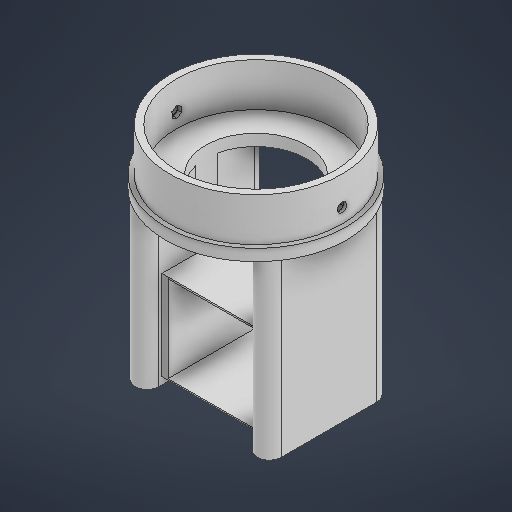
# Autodesk Inventor part: cam_mount0
Saved by Autodesk Inventor 2027 (Build 310192060, 192F)
## iProperties
Created: 2026-07-16
Part Number: cam_mount0
Material: Generic
Document SubType Name: Modeling
Designer: farde
Density: 1 g/cm^3
Appearance: Default
Author: farde
Autodesk Inventor part; units mm, degrees
ref_plane "YZ Plane" through (0, 0, 0) normal (1, 0, 0) x (0, 1, 0)
ref_plane "XZ Plane" through (0, 0, 0) normal (0, 1, 0) x (-1, 0, 0)
ref_plane "XY Plane" through (0, 0, 0) normal (0, 0, 1) x (1, 0, 0)
sketch "Sketch1" plane through (0, 0, 0) normal (0, 1, 0) x (-1, 0, 0)
  circle A0 centre (0, 0) radius 29.85
  circle A1 centre (0, 0) radius 27.5
  dimension "d0" = 59.7
  dimension "d1" = 55
  constraints: 2 centre point, 2 coincident
  measures "d0" diameter of A0
  measures "d1" diameter of A1
extrude "Extrusion1" add sketch "Sketch1" along normal blind 15
sketch "Sketch2" plane through (0, 0, 0) normal (0, 1, 0) x (-1, 0, 0)
  circle A0 centre (0, 0) radius 31.4135
  circle A1 centre (0, 0) radius 28.9404
  circle A2 centre (0, 0) radius 31.4135
  circle A3 centre (0, 0) radius 20.0919
  dimension "d6" = 40.1837
  constraints: 4 centre point, 4 coincident, 1 concentric
  measures "d6" diameter of A3
extrude "Extrusion2" add sketch "Sketch2" against normal blind 4 contours A0 | A1 | A3
sketch "Sketch3" plane through (0, -4, 0) normal (0, -1, 0) x (1, 0, 0)
  line L0 (21.2066, 16.5968) -> (21.2066, -16.5968) construction
  line L1 (17.0959, 16.5968) -> (17.0959, -16.5968)
  line L2 (25.3174, -16.5968) -> (25.3174, 16.5968)
  arc A0 (25.3174, 16.5968) -> (17.0959, 16.5968) centre (21.2066, 16.5968) ccw
  arc A1 (17.0959, -16.5968) -> (25.3174, -16.5968) centre (21.2066, -16.5968) ccw
  point P0 (0, 0)
  point P1 (21.2066, 0)
  dimension "d28" = 8.2215
  constraints: 8 end point, 4 point on circle, 4 tangent, 2 centre point, 1 midpoint, 1 parallel, 1 vertical
  measures "d28" distance between parallel lines of L1 L2
extrude "Extrusion3" add sketch "Sketch3" along normal blind 60
mirror "Mirror1" about plane through (0, 0, 0) normal (1, 0, 0) of "Extrusion3"
sketch "Sketch4" plane through (0, 0, 0) normal (0, 1, 0) x (1, 0, 0)
  circle A0 centre (0, 0) radius 17.5
  dimension "d11" = 35
  constraints: 1 centre point, 1 coincident
  measures "d11" diameter of A0
extrude "Extrusion4" cut sketch "Sketch4" against normal blind 60
sketch "Sketch5" plane through (17.0959, -64, -16.5968) normal (-1, 0, 0) x (0, 0, 1)
  line L0 (32.0968, 2.4749) -> (1.0968, 2.4749)
  line L1 (1.0968, 2.4749) -> (1.0968, 33.4749)
  line L2 (1.0968, 33.4749) -> (32.0968, 33.4749)
  line L3 (32.0968, 33.4749) -> (32.0968, 2.4749)
  line L4 (32.0968, 2.4749) -> (1.0968, 33.4749) construction
  line L5 (1.0968, 2.4749) -> (32.0968, 33.4749) construction
  point P0 (16.5968, 64)
  point P1 (16.5968, 17.9749)
  dimension "d12" = 31
  dimension "d13" = 31
  constraints: 12 end point, 2 midpoint, 2 parallel, 1 horizontal, 1 perpendicular
  measures "d12" distance of L1.end L2.end
  measures "d13" distance of L0.end L1.end
extrude "Extrusion5" add sketch "Sketch5" along normal blind 36.1875
sketch "Sketch6" plane through (17.0959, -61.5251, -15.5) normal (0, -1, 0) x (1, 0, 0)
  point P0 (-17.0959, 15.5)
sketch "Sketch8" plane through (-25.3174, -64, -16.5968) normal (-1, 0, 0) x (0, 0, 1)
  line L0 (22.3596, 21.0912) -> (-66.3415, 21.0912) construction
  line L1 (-66.3415, 21.0912) -> (-66.3415, 85.9745) construction
  line L2 (-66.3415, 85.9745) -> (22.3596, 85.9745) construction
  line L3 (22.3596, 85.9745) -> (22.3596, 21.0912) construction
  spline S0 degree 2 poles (14.1923, 27.2024) (14.1923, 30.3627) (16.0295, 33.3231) (17.9428, 33.3231) knots 0 0 0 1 2 2 2
  spline S1 degree 2 poles (17.9428, 33.3231) (19.8847, 33.3231) (21.7028, 30.3056) (21.7028, 27.2119) knots 0 0 0 1 2 2 2
  spline S2 degree 2 poles (21.7028, 27.2119) (21.7028, 24.0326) (19.8656, 21.0912) (17.9428, 21.0912) knots 0 0 0 1 2 2 2
  spline S3 degree 2 poles (17.9428, 21.0912) (16.0104, 21.0912) (14.1923, 24.1373) (14.1923, 27.2024) knots 0 0 0 1 2 2 2
  spline S4 degree 2 poles (16.2103, 30.7816) (15.9819, 30.2009) (15.7915, 28.4113) (15.7915, 27.2024) knots 0 0 0 1 2 2 2
  spline S5 degree 2 poles (15.7915, 27.2024) (15.7915, 25.9935) (15.9819, 24.2134) (16.2199, 23.6137) knots 0 0 0 1 2 2 2
  spline S6 degree 2 poles (16.2199, 23.6137) (16.4578, 23.0141) (17.286, 22.3953) (17.9428, 22.3953) knots 0 0 0 1 2 2 2
  spline S7 degree 2 poles (17.9428, 22.3953) (18.5996, 22.3953) (19.4468, 23.0141) (19.6943, 23.6328) knots 0 0 0 1 2 2 2
  spline S8 degree 2 poles (19.6943, 23.6328) (19.9323, 24.2325) (20.1036, 26.0601) (20.1036, 27.2119) knots 0 0 0 1 2 2 2
  spline S9 degree 2 poles (20.1036, 27.2119) (20.1036, 28.4494) (19.9513, 30.1057) (19.7038, 30.753) knots 0 0 0 1 2 2 2
  spline S10 degree 2 poles (19.7038, 30.753) (19.4754, 31.3622) (18.6282, 32.019) (17.9428, 32.019) knots 0 0 0 1 2 2 2
  spline S11 degree 2 poles (17.9428, 32.019) (17.2955, 32.019) (16.4483, 31.4003) (16.2103, 30.7816) knots 0 0 0 1 2 2 2
  spline S12 degree 2 poles (6.7389, 24.1278) (6.7389, 25.3938) (8.4714, 27.1263) (9.7374, 27.1263) knots 0 0 0 1 2 2 2
  spline S13 degree 2 poles (9.7374, 27.1263) (10.9939, 27.1263) (12.7454, 25.4033) (12.7454, 24.1278) knots 0 0 0 1 2 2 2
  spline S14 degree 2 poles (12.7454, 24.1278) (12.7454, 22.8617) (11.013, 21.1293) (9.7374, 21.1293) knots 0 0 0 1 2 2 2
  spline S15 degree 2 poles (9.7374, 21.1293) (8.4714, 21.1293) (6.7389, 22.8617) (6.7389, 24.1278) knots 0 0 0 1 2 2 2
  spline S16 degree 2 poles (7.9764, 24.1278) (7.9764, 23.3663) (8.9854, 22.3287) (9.7374, 22.3287) knots 0 0 0 1 2 2 2
  spline S17 degree 2 poles (9.7374, 22.3287) (10.4989, 22.3287) (11.5079, 23.3663) (11.5079, 24.1278) knots 0 0 0 1 2 2 2
  spline S18 degree 2 poles (11.5079, 24.1278) (11.5079, 24.8988) (10.4799, 25.9269) (9.7374, 25.9269) knots 0 0 0 1 2 2 2
  spline S19 degree 2 poles (9.7374, 25.9269) (8.9854, 25.9269) (7.9764, 24.8798) (7.9764, 24.1278) knots 0 0 0 1 2 2 2
  point P0 (16.5968, 64)
  constraints: 2 other
sketch "Sketch9" plane through (0, 0, 0) normal (1, 0, 0) x (0, 1, 0)
  circle A0 centre (5, 0) radius 1.6
  line L0 (0, -31.4135) -> (0, 31.4135) projected
  point P0 (0, 0)
  dimension "d22" = 3.2
  dimension "d25" = 5
  constraints: 1 centre point
  measures "d22" diameter of A0
  measures "d25" distance from line of L0 A0.centre
extrude "Extrusion8" cut sketch "Sketch9" along normal mid plane 78.2
sketch "Sketch10" plane through (0, 0, 0) normal (1, 0, 0) x (0, 1, 0)
  line L0 (5.9683, -1.6274) -> (4.0574, -1.6823)
  line L1 (4.0574, -1.6823) -> (3.0544, -0.0549)
  line L2 (3.0544, -0.0549) -> (3.9623, 1.6274)
  line L3 (3.9623, 1.6274) -> (5.8731, 1.6823)
  line L4 (5.8731, 1.6823) -> (6.8761, 0.0549)
  line L5 (6.8761, 0.0549) -> (5.9683, -1.6274)
  point P0 (0, 0)
  point P1 (4.9653, 0)
  constraints: 12 end point, 13 other
extrude "Extrusion9" cut sketch "Sketch10" along normal mid plane 57.5625
sketch "Sketch11" plane through (-25.3174, -64, -16.5968) normal (-1, 0, 0) x (0, 0, 1)
  line L0 (23.7481, 35.1884) -> (-5.73, 35.1884) construction
  line L1 (-5.73, 35.1884) -> (-5.73, 39.6022) construction
  line L2 (-5.73, 39.6022) -> (23.7481, 39.6022) construction
  line L3 (23.7481, 39.6022) -> (23.7481, 35.1884) construction
  line L4 (21.6116, 35.7812) -> (22.9306, 38.3722)
  line L5 (22.9306, 38.3722) -> (23.3653, 38.3722)
  line L6 (23.3653, 38.3722) -> (21.9722, 35.6824)
  line L7 (21.9722, 35.6824) -> (23.5456, 35.6824)
  line L8 (23.5456, 35.6824) -> (23.5456, 35.3242)
  line L9 (23.5456, 35.3242) -> (21.6116, 35.3242)
  line L10 (21.6116, 35.3242) -> (21.6116, 35.7812)
  line L11 (19.9715, 35.1884) -> (21.1645, 39.0342)
  line L12 (21.1645, 39.0342) -> (21.5103, 39.0342)
  line L13 (21.5103, 39.0342) -> (20.3222, 35.1884)
  line L14 (20.3222, 35.1884) -> (19.9715, 35.1884)
  line L15 (17.7559, 38.3722) -> (19.6356, 38.3722)
  line L16 (19.6356, 38.3722) -> (19.6356, 37.94)
  spline S0 degree 2 poles (19.6356, 37.94) (19.433, 37.7498) (19.0724, 37.3966) (18.8995, 37.2064) knots 0 0 0 1 2 2 2
  spline S1 degree 2 poles (18.8995, 37.2064) (18.5512, 36.8235) (18.2968, 36.3641) (18.2968, 36.1196) knots 0 0 0 1 2 2 2
  spline S2 degree 2 poles (18.2968, 36.1196) (18.2968, 35.9911) (18.3759, 35.7985) (18.4475, 35.7367) knots 0 0 0 1 2 2 2
  spline S3 degree 2 poles (18.4475, 35.7367) (18.5191, 35.675) (18.7068, 35.6132) (18.8205, 35.6132) knots 0 0 0 1 2 2 2
  spline S4 degree 2 poles (18.8205, 35.6132) (18.9291, 35.6132) (19.1514, 35.6676) (19.2527, 35.7096) knots 0 0 0 1 2 2 2
  spline S5 degree 2 poles (19.2527, 35.7096) (19.3392, 35.7441) (19.4997, 35.8429) (19.5491, 35.8775) knots 0 0 0 1 2 2 2
  line L17 (19.5491, 35.8775) -> (19.5713, 35.8775)
  line L18 (19.5713, 35.8775) -> (19.5713, 35.4428)
  spline S6 degree 2 poles (19.5713, 35.4428) (19.4454, 35.381) (18.9934, 35.26) (18.7908, 35.26) knots 0 0 0 1 2 2 2
  spline S7 degree 2 poles (18.7908, 35.26) (18.3635, 35.26) (17.8819, 35.712) (17.8819, 36.0973) knots 0 0 0 1 2 2 2
  spline S8 degree 2 poles (17.8819, 36.0973) (17.8819, 36.2777) (17.9658, 36.579) (18.0399, 36.7074) knots 0 0 0 1 2 2 2
  spline S9 degree 2 poles (18.0399, 36.7074) (18.114, 36.8408) (18.3289, 37.1026) (18.4475, 37.2286) knots 0 0 0 1 2 2 2
  spline S10 degree 2 poles (18.4475, 37.2286) (18.6401, 37.4386) (19.1119, 37.8881) (19.2527, 38.019) knots 0 0 0 1 2 2 2
  line L19 (19.2527, 38.019) -> (17.7559, 38.019)
  line L20 (17.7559, 38.019) -> (17.7559, 38.3722)
  spline S11 degree 2 poles (15.4514, 36.8482) (15.4514, 37.6683) (15.9281, 38.4365) (16.4245, 38.4365) knots 0 0 0 1 2 2 2
  spline S12 degree 2 poles (16.4245, 38.4365) (16.9284, 38.4365) (17.4002, 37.6535) (17.4002, 36.8507) knots 0 0 0 1 2 2 2
  spline S13 degree 2 poles (17.4002, 36.8507) (17.4002, 36.0257) (16.9235, 35.2625) (16.4245, 35.2625) knots 0 0 0 1 2 2 2
  spline S14 degree 2 poles (16.4245, 35.2625) (15.9231, 35.2625) (15.4514, 36.0529) (15.4514, 36.8482) knots 0 0 0 1 2 2 2
  spline S15 degree 2 poles (15.975, 37.777) (15.9157, 37.6263) (15.8663, 37.1619) (15.8663, 36.8482) knots 0 0 0 1 2 2 2
  spline S16 degree 2 poles (15.8663, 36.8482) (15.8663, 36.5345) (15.9157, 36.0726) (15.9775, 35.917) knots 0 0 0 1 2 2 2
  spline S17 degree 2 poles (15.9775, 35.917) (16.0392, 35.7614) (16.2541, 35.6009) (16.4245, 35.6009) knots 0 0 0 1 2 2 2
  spline S18 degree 2 poles (16.4245, 35.6009) (16.595, 35.6009) (16.8148, 35.7614) (16.879, 35.922) knots 0 0 0 1 2 2 2
  spline S19 degree 2 poles (16.879, 35.922) (16.9408, 36.0776) (16.9852, 36.5518) (16.9852, 36.8507) knots 0 0 0 1 2 2 2
  spline S20 degree 2 poles (16.9852, 36.8507) (16.9852, 37.1718) (16.9457, 37.6016) (16.8815, 37.7695) knots 0 0 0 1 2 2 2
  spline S21 degree 2 poles (16.8815, 37.7695) (16.8222, 37.9276) (16.6024, 38.0981) (16.4245, 38.0981) knots 0 0 0 1 2 2 2
  spline S22 degree 2 poles (16.4245, 38.0981) (16.2566, 38.0981) (16.0367, 37.9375) (15.975, 37.777) knots 0 0 0 1 2 2 2
  line L21 (13.794, 35.1884) -> (14.987, 39.0342)
  line L22 (14.987, 39.0342) -> (15.3328, 39.0342)
  line L23 (15.3328, 39.0342) -> (14.1447, 35.1884)
  line L24 (14.1447, 35.1884) -> (13.794, 35.1884)
  line L25 (11.5784, 38.3722) -> (13.4581, 38.3722)
  line L26 (13.4581, 38.3722) -> (13.4581, 37.94)
  spline S23 degree 2 poles (13.4581, 37.94) (13.2555, 37.7498) (12.8949, 37.3966) (12.722, 37.2064) knots 0 0 0 1 2 2 2
  spline S24 degree 2 poles (12.722, 37.2064) (12.3737, 36.8235) (12.1193, 36.3641) (12.1193, 36.1196) knots 0 0 0 1 2 2 2
  spline S25 degree 2 poles (12.1193, 36.1196) (12.1193, 35.9911) (12.1983, 35.7985) (12.27, 35.7367) knots 0 0 0 1 2 2 2
  spline S26 degree 2 poles (12.27, 35.7367) (12.3416, 35.675) (12.5293, 35.6132) (12.6429, 35.6132) knots 0 0 0 1 2 2 2
  spline S27 degree 2 poles (12.6429, 35.6132) (12.7516, 35.6132) (12.9739, 35.6676) (13.0752, 35.7096) knots 0 0 0 1 2 2 2
  spline S28 degree 2 poles (13.0752, 35.7096) (13.1616, 35.7441) (13.3222, 35.8429) (13.3716, 35.8775) knots 0 0 0 1 2 2 2
  line L27 (13.3716, 35.8775) -> (13.3938, 35.8775)
  line L28 (13.3938, 35.8775) -> (13.3938, 35.4428)
  spline S29 degree 2 poles (13.3938, 35.4428) (13.2679, 35.381) (12.8158, 35.26) (12.6133, 35.26) knots 0 0 0 1 2 2 2
  spline S30 degree 2 poles (12.6133, 35.26) (12.186, 35.26) (11.7043, 35.712) (11.7043, 36.0973) knots 0 0 0 1 2 2 2
  spline S31 degree 2 poles (11.7043, 36.0973) (11.7043, 36.2777) (11.7883, 36.579) (11.8624, 36.7074) knots 0 0 0 1 2 2 2
  spline S32 degree 2 poles (11.8624, 36.7074) (11.9365, 36.8408) (12.1514, 37.1026) (12.27, 37.2286) knots 0 0 0 1 2 2 2
  spline S33 degree 2 poles (12.27, 37.2286) (12.4626, 37.4386) (12.9344, 37.8881) (13.0752, 38.019) knots 0 0 0 1 2 2 2
  line L29 (13.0752, 38.019) -> (11.5784, 38.019)
  line L30 (11.5784, 38.019) -> (11.5784, 38.3722)
  spline S34 degree 2 poles (9.2442, 37.3842) (9.2442, 37.6189) (9.3998, 38.0165) (9.5307, 38.1499) knots 0 0 0 1 2 2 2
  spline S35 degree 2 poles (9.5307, 38.1499) (9.6666, 38.2907) (10.0074, 38.4365) (10.2125, 38.4365) knots 0 0 0 1 2 2 2
  spline S36 degree 2 poles (10.2125, 38.4365) (10.4175, 38.4365) (10.7559, 38.2981) (10.8843, 38.1598) knots 0 0 0 1 2 2 2
  spline S37 degree 2 poles (10.8843, 38.1598) (11.0424, 37.9943) (11.2202, 37.4386) (11.2202, 37.0335) knots 0 0 0 1 2 2 2
  spline S38 degree 2 poles (11.2202, 37.0335) (11.2202, 36.6358) (11.0572, 35.9961) (10.8868, 35.759) knots 0 0 0 1 2 2 2
  spline S39 degree 2 poles (10.8868, 35.759) (10.7213, 35.5268) (10.1976, 35.2674) (9.8543, 35.2674) knots 0 0 0 1 2 2 2
  spline S40 degree 2 poles (9.8543, 35.2674) (9.753, 35.2674) (9.5752, 35.2872) (9.5085, 35.3094) knots 0 0 0 1 2 2 2
  line L31 (9.5085, 35.3094) -> (9.5085, 35.7021)
  line L32 (9.5085, 35.7021) -> (9.5258, 35.7021)
  spline S41 degree 2 poles (9.5258, 35.7021) (9.5826, 35.6725) (9.7901, 35.6206) (9.9086, 35.6206) knots 0 0 0 1 2 2 2
  spline S42 degree 2 poles (9.9086, 35.6206) (10.289, 35.6206) (10.7559, 36.1344) (10.8003, 36.6383) knots 0 0 0 1 2 2 2
  spline S43 degree 2 poles (10.8003, 36.6383) (10.6546, 36.537) (10.3483, 36.4259) (10.1655, 36.4259) knots 0 0 0 1 2 2 2
  spline S44 degree 2 poles (10.1655, 36.4259) (9.9877, 36.4259) (9.7209, 36.4975) (9.5752, 36.6062) knots 0 0 0 1 2 2 2
  spline S45 degree 2 poles (9.5752, 36.6062) (9.4072, 36.7321) (9.2442, 37.1224) (9.2442, 37.3842) knots 0 0 0 1 2 2 2
  spline S46 degree 2 poles (9.6592, 37.4015) (9.6592, 37.2138) (9.758, 36.9594) (9.8666, 36.8705) knots 0 0 0 1 2 2 2
  spline S47 degree 2 poles (9.8666, 36.8705) (9.9482, 36.8062) (10.1507, 36.7642) (10.2569, 36.7642) knots 0 0 0 1 2 2 2
  spline S48 degree 2 poles (10.2569, 36.7642) (10.4002, 36.7642) (10.6694, 36.8507) (10.8003, 36.9322) knots 0 0 0 1 2 2 2
  spline S49 degree 2 poles (10.8003, 36.9322) (10.8028, 36.9767) (10.8077, 37.0607) (10.8077, 37.1249) knots 0 0 0 1 2 2 2
  spline S50 degree 2 poles (10.8077, 37.1249) (10.8077, 37.441) (10.6842, 37.8288) (10.5904, 37.9301) knots 0 0 0 1 2 2 2
  spline S51 degree 2 poles (10.5904, 37.9301) (10.5039, 38.0264) (10.3162, 38.103) (10.21, 38.103) knots 0 0 0 1 2 2 2
  spline S52 degree 2 poles (10.21, 38.103) (9.963, 38.103) (9.6592, 37.7523) (9.6592, 37.4015) knots 0 0 0 1 2 2 2
  point P0 (16.5968, 64)
  constraints: 2 other
emboss "Emboss1" sketch "Sketch11" operation add depth 1 direction (1, 0, 0)
emboss "Emboss3" sketch "Sketch8" operation add depth 1 direction (1, 0, 0)
sketch "Sketch12" plane through (17.0959, -61.5251, -15.5) normal (0, 0, -1) x (-1, 0, 0)
  line L0 (2.0959, 30.4399) -> (32.0959, 30.4399)
  line L1 (32.0959, 30.4399) -> (32.0959, 0.4399)
  line L2 (32.0959, 0.4399) -> (2.0959, 0.4399)
  line L3 (2.0959, 0.4399) -> (2.0959, 30.4399)
  line L4 (2.0959, 30.4399) -> (32.0959, 0.4399) construction
  line L5 (32.0959, 30.4399) -> (2.0959, 0.4399) construction
  point P0 (17.0959, 61.5251)
  point P1 (17.0959, 15.4399)
  dimension "d35" = 30
  dimension "d36" = 30
  constraints: 12 end point, 2 midpoint, 2 parallel, 1 horizontal, 1 perpendicular
  measures "d35" distance of L1.end L2.end
  measures "d36" distance of L0.end L1.end
extrude "Extrusion10" cut sketch "Sketch12" against normal blind 33.8125
body "Solid1"
